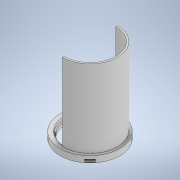
# Autodesk Inventor part: Kessil holder
Saved by Autodesk Inventor 2022 (Build 260153000, 153)
## iProperties
Created: 2023-03-20
Part Number: Kessil holder
Material: Generic
Document SubType Name: Modeling
Designer: tmass
Density: 1 g/cm^3
Appearance: Default
Author: tmass
Autodesk Inventor part; units mm, degrees
ref_plane "YZ Plane" through (0, 0, 0) normal (1, 0, 0) x (0, 1, 0)
ref_plane "XZ Plane" through (0, 0, 0) normal (0, 1, 0) x (-1, 0, 0)
ref_plane "XY Plane" through (0, 0, 0) normal (0, 0, 1) x (1, 0, 0)
sketch "Sketch1" plane through (0, 0, 0) normal (0, 1, 0) x (-1, 0, 0)
  circle A0 centre (0, 0) radius 32
  circle A1 centre (0, 0) radius 34
  circle A2 centre (0, 0) radius 30
  line L0 (0, 34) -> (0, 32)
  line L1 (0, -32) -> (0, -34)
  dimension "d0" = 64
  dimension "d1" = 2
  dimension "d2" = 2
  constraints: 4 end point, 4 point on circle, 3 centre point, 3 coincident, 2 point on line, 1 vertical
  measures "d0" diameter of A0
  measures "d1" radial gap between concentric circles of A1 A0
  measures "d2" radial gap between concentric circles of A2 A0
extrude "Extrusion1" add sketch "Sketch1" along normal blind 100 contours A0 L1 A1 L0 picked at (-2.7122, -33.004)
sketch "Sketch2" plane through (0, 0, 0) normal (0, 1, 0) x (-1, 0, 0)
  circle A0 centre (0, 0) radius 30 projected
  circle A1 centre (0, 0) radius 32 projected
extrude "Extrusion2" add sketch "Sketch2" against normal blind 4
sketch "Sketch3" plane through (0, 0, 0) normal (0, 1, 0) x (-1, 0, 0)
  circle A0 centre (0, 0) radius 37
  arc A1 (0, -32) -> (0, 32) centre (0, 0) ccw projected
  circle A2 centre (0, 0) radius 30 projected
  circle A3 centre (0, 0) radius 32
  point P0 (0, 32)
  dimension "d7" = 74
  constraints: 2 centre point, 2 coincident, 1 concentric
  measures "d7" diameter of A0
extrude "Extrusion3" add sketch "Sketch3" along normal mid plane 8 contours A0
sketch "Sketch4" plane through (0, 0, 0) normal (0, 1, 0) x (-1, 0, 0)
  circle A0 centre (24, 24) radius 5.5
  circle A1 centre (0, 0) radius 30 projected
  line L0 (48.965, 0) -> (-22.6719, 0) construction
  circle A2 centre (0, 0) radius 37 projected
  line L1 (24, 24) -> (0, 0) construction
  circle A3 centre (-24, 24) radius 5.5
  circle A4 centre (-24, -24) radius 5.5
  circle A5 centre (24, -24) radius 5.5
  point P0 (22.5777, 29.3129)
  point P1 (29.3129, 22.5777)
  dimension "d10" = 11
  dimension "d11" = 45
  dimension "d16" = 24
  dimension "d19" = 360
  constraints: 4 centre point, 4 end point, 1 horizontal, 9 other
  measures "d10" diameter of A0
  measures "d11" angle of L0 L1
  measures "d16" horizontal distance of point (0, 0) L1.start
extrude "Extrusion6" cut sketch "Sketch4" against normal blind 3.5 contours A0 A2 | A2 A0 A1 | A1 A0 | A3 A1 A2 | A2 A3 | A3 A1 | A5 A2 | A2 A5 A1 | A4 A1 A2 | A2 A4 | A1 A5 | A4 A1
body "Solid1"
